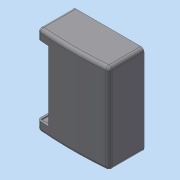
# Autodesk Inventor part: cuerpo
Saved by Autodesk Inventor 2013 (Build 170138000, 138)
## iProperties
Created: 2017-05-15
Part Number: cuerpo
Material: Generic
Document SubType Name: Modeling
Designer: Fede
Density: 1 g/cm^3
Author: Fede
Autodesk Inventor part; units mm, degrees
ref_plane "YZ Plane" through (0, 0, 0) normal (1, 0, 0) x (0, 1, 0)
ref_plane "XZ Plane" through (0, 0, 0) normal (0, 1, 0) x (-1, 0, 0)
ref_plane "XY Plane" through (0, 0, 0) normal (0, 0, 1) x (1, 0, 0)
sketch "Sketch1" plane through (0, 0, 0) normal (0, 1, 0) x (-1, 0, 0)
  line L0 (-18.5654, 9.2536) -> (2.9346, 9.2536)
  line L1 (2.9346, 9.2536) -> (2.9346, -17.7464)
  line L2 (2.9346, -17.7464) -> (-18.5654, -17.7464)
  line L3 (-18.5654, -17.7464) -> (-18.5654, 9.2536)
  circle A0 centre (-15.5654, 6.2536) radius 0.875
  line L4 (-17.5654, 3.454) -> (-17.5654, -16.6136)
  line L5 (2.9346, 8.2536) -> (-13.3293, 8.2536)
  line L6 (-17.5654, 3.454) -> (-17.5654, 4.0175)
  line L7 (-17.5654, -16.6136) -> (-17.5654, -17.7464)
  arc A1 (-17.5654, 4.0175) -> (-13.3293, 8.2536) centre (-15.5654, 6.2536) ccw
  point P0 (0, 0)
  dimension "d0" = 21.5
  dimension "d2" = 27
  dimension "d3" = 3
  dimension "d4" = 3
  dimension "d6" = 1.75
  dimension "d7" = 1
  dimension "d8" = 1
  constraints: 16 end point, 3 parallel, 2 centre point, 2 perpendicular, 2 point on circle, 2 point on line, 1 coincident, 1 collinear, 1 horizontal
  measures "d0" distance of L0.start L0.end
  measures "d2" distance of L2.end L0.start
  measures "d3" distance from line of A1.centre L3
  measures "d4" distance from line of A1.centre L0
  measures "d6" diameter of A0
  measures "d7" distance between parallel lines of L0 L5
  measures "d8" distance between parallel lines of L3 L4
extrude "Extrusion1" add sketch "Sketch1" along normal blind 20 contours L0 L1 L5 A1 L6 L4 L7 L2 L3
sketch "Sketch2" plane through (0, 0, 0) normal (0, -1, 0) x (1, 0, 0)
  line L0 (18.5654, 9.2536) -> (-2.9346, 9.2536)
  line L1 (-2.9346, 9.2536) -> (-2.9346, -17.7464)
  line L2 (-2.9346, -17.7464) -> (18.5654, -17.7464)
  line L3 (18.5654, -17.7464) -> (18.5654, 9.2536)
  point P0 (0, 0)
  constraints: 8 end point, 2 parallel, 1 horizontal, 1 perpendicular
extrude "Extrusion2" add sketch "Sketch2" along normal blind 1
mirror "Mirror1" about plane through (18.5654, 0, -17.7464) normal (0, 0, -1) of "Extrusion1", "Extrusion2"
mirror "Mirror2" about plane through (-2.9346, 0, 8.2536) normal (-1, 0, 0) of "Extrusion1", "Extrusion2", "Mirror1"
sketch "Sketch3" plane through (18.5654, -1, 9.2536) normal (0, 0, 1) x (1, 0, 0)
  line L0 (0, 0) -> (-43, 0) projected
  arc A0 (-43, 0) -> (0, 0) centre (-21.5, 230.625) ccw
  line L1 (-40.8006, -1) -> (-1.6118, -1)
  point P0 (-18.5654, 1)
  dimension "d13" = 1
  constraints: 2 end point, 2 point on circle, 1 centre point, 1 parallel, 1 tangent
  measures "d13" distance between parallel lines of L0 L1
extrude "Extrusion3" add sketch "Sketch3" against normal blind 54
fillet "Fillet1" radius 2 8 edges at (-24.4346, -1, -17.7464) (-2.9346, -2, -44.7464) (-24.4346, 9.5, -44.7464) (18.5654, 9.5, -44.7464) (-24.4346, 9.5, 9.2536) (-2.9346, -2, 9.2536) (18.5654, 9.5, 9.2536) (18.5654, -1, -17.7464)
sketch "Sketch4" plane through (0, 0, 0) normal (0, 1, 0) x (1, 0, 0)
  line L0 (-38.0807, 38.7464) -> (-17.4346, 38.7464)
  line L1 (-17.4346, 38.7464) -> (-17.4346, -3.2536)
  line L2 (-17.4346, -3.2536) -> (-38.0807, -3.2536)
  line L3 (-38.0807, -3.2536) -> (-38.0807, 38.7464)
  line L4 (-24.4346, 42.7464) -> (-24.4346, -7.2536) projected
  arc A0 (-23.4346, 39.5104) -> (-19.1985, 43.7464) centre (-21.4346, 41.7464) ccw projected
  arc A1 (-19.1985, -8.2536) -> (-23.4346, -4.0175) centre (-21.4346, -6.2536) ccw projected
  point P0 (0, 0)
  dimension "d17" = 7
  constraints: 8 end point, 2 parallel, 2 tangent, 1 horizontal, 1 perpendicular
  measures "d17" distance between parallel lines of L1 L4
extrude "Extrusion4" cut sketch "Sketch4" along normal mid plane 50
body "Solid1"
